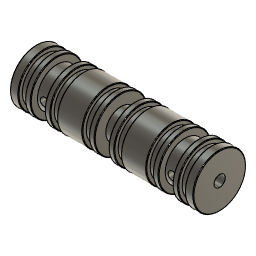
Timer ORings v3 (Autodesk Fusion 360 design; units mm, degrees)
Autodesk Fusion 360 part; units mm, degrees
sketch "Piston" plane through (0, 0, 0) normal (0, 1, 0) x (1, 0, 0)
  line L0 (0, 0) -> (0, -9.398)
  line L1 (0, -9.398) -> (1, -9.398)
  line L2 (1, -9.398) -> (2.5527, -9.398) construction
  line L3 (7.3876, -9.398) -> (7.3876, -7)
  line L4 (7.3876, -7) -> (12.3876, -7)
  line L5 (12.3876, -7) -> (12.3876, -9.398)
  line L6 (12.3876, -9.398) -> (14.3876, -9.398)
  line L7 (14.3876, -9.398) -> (14.3876, -7.9883)
  line L8 (14.3876, -7.9883) -> (16.7752, -7.9883)
  line L9 (16.7752, -7.9883) -> (16.7752, -9.398)
  line L10 (-1.3, -9.525) -> (30.7127, -9.525)
  line L11 (25.7752, -9.398) -> (25.7752, -7.9883)
  line L12 (25.7752, -7.9883) -> (28.1628, -7.9883)
  line L13 (28.1628, -7.9883) -> (28.1628, -9.398)
  line L14 (30.1628, -9.398) -> (30.1628, -5.398)
  line L15 (30.1628, -5.398) -> (32.6628, -5.398)
  line L16 (35.1628, -5.398) -> (35.1628, -9.398)
  line L17 (-1.7467, -7.9883) -> (1, -7.9883) construction
  line L18 (5.3876, -9.398) -> (5.3876, -7.9883)
  line L19 (5.3876, -7.9883) -> (3, -7.9883)
  line L20 (3, -7.9883) -> (3, -9.398)
  line L21 (32.6628, 7.102) -> (32.6628, -15.898)
  line L22 (16.7752, -9.398) -> (25.7752, -9.398)
  line L23 (28.1628, -9.398) -> (30.1628, -9.398)
  line L24 (5.3876, -9.398) -> (7.3876, -9.398)
  line L25 (3, -9.398) -> (0, -9.398)
  line L26 (32.6628, -5.398) -> (35.1628, -5.398)
  line L27 (0, 0) -> (32.6628, 0)
  line L28 (0, -2) -> (12, -2)
  line L29 (12, -2) -> (12, 0)
  dimension "d75" = 9.398
  dimension "d77" = 2.3876
  dimension "d78" = 9.525
  dimension "d79" = 2
  dimension "d80" = 5
  dimension "d81" = 9
  dimension "d82" = 2.3876
  dimension "d83" = 4
  dimension "d84" = 5
  dimension "d85" = 7.9883
  dimension "d86" = 2
  dimension "d87" = 2.3876
  dimension "d88" = 2
  dimension "d90" = 11.3876
  dimension "d91" = 3
  dimension "d92" = 2
  constraint coincident L0.start L27.start
  constraint vertical L0
  constraint perpendicular L0 L1
  constraint perpendicular L0 L2
  constraint coincident L2 L3.start
  constraint perpendicular L2 L3
  constraint perpendicular L3 L4
  constraint coincident L2 L5.end
  constraint perpendicular L2 L5
  constraint coincident L2 L6.end
  constraint perpendicular L6 L7
  constraint perpendicular L7 L8
  constraint coincident L2 L9.end
  constraint perpendicular L2 L9
  constraint parallel L2 L10
  constraint coincident L2 L11.start
  constraint perpendicular L2 L11
  constraint perpendicular L11 L12
  constraint coincident L2 L13.end
  constraint perpendicular L2 L13
  constraint coincident L2 L14.start
  constraint perpendicular L14 L15
  constraint coincident L2 L16.end
  constraint perpendicular L2 L16
  constraint perpendicular L5 L17
  constraint coincident L17 L18.end
  constraint perpendicular L17 L18
  constraint coincident L17 L19.end
  constraint perpendicular L2 L20
  constraint collinear L8 L17
  constraint perpendicular L2 L21
  constraint perpendicular L3 L24
  constraint perpendicular L0 L25
  constraint coincident L21 L15.end
  constraint perpendicular L14 L26
  constraint coincident L21 L27.end
  constraint perpendicular L21 L27
  constraint collinear L12 L17
  constraint coincident L0 L28.start
  constraint perpendicular L0 L28
  constraint coincident L27 L29.end
  constraint perpendicular L27 L29
  measures "d75" distance of L0.start L0.end
  measures "d77" distance of L7 L9
  measures "d78" distance of L0.start L10
  measures "d79" distance of L5 L7
  measures "d80" distance of L3 L5
  measures "d81" distance of L9 L11
  measures "d82" distance of L11 L13
  measures "d83" distance of L14.start L14.end
  measures "d84" distance of L14.end L16.start
  measures "d85" distance of L0.start L17
  measures "d86" distance of L3 L18
  measures "d87" distance of L18 L20
  measures "d88" distance of L13 L14
  measures "d90" distance of L7.end L19.end
  measures "d91" distance of L0 L20
  measures "d92" distance of L27 L28
revolve "Revolve3" add sketch "Piston" angle 360 about axis through (0, 0, 0) along (1, 0, 0) contours L0 L1 L3 L4 L5 L6 L7 L8 L9 L11 L12 L13 L14 L15 L18 L19 L20 L21 L22 L23 L24 L25 L27 L28 L29 makes body 1
sketch "Sketch6" plane through (0, 0, 0) normal (0, 1, 0) x (1, 0, 0)
  line L0 (7.3876, -7) -> (12.3876, -7)
  circle A0 centre (9.8876, 0) radius 1.5
  line L1 (9.8876, -19.5) -> (9.8876, 5.5) construction
  dimension "d96" = 3
  constraint vertical L1
  constraint midpoint L0 L1
  constraint coincident A0.centre L1
  measures "d96" diameter of A0
extrude "Extrude15" cut sketch "Sketch6" along normal through all and the other way through all bodies 1
mirror "Mirror1" about plane through (32.6628, 0, 0) normal (1, 0, 0) of bodies 1 makes body 2
combine "Combine3" operation add target body 1 tool bodies 2
fillet "Fillet2" radius 0.2 20 edges at (0, -3.3985, -8.762) (3, -3.3985, -8.762) (5.3876, -3.3985, -8.762) (7.3876, -3.3985, -8.762) (12.3876, -3.3985, -8.762) (14.3876, -3.3985, -8.762) (16.7752, -3.3985, -8.762) (25.7752, -3.3985, -8.762) (28.1628, -3.3985, -8.762) (37.1628, -3.3985, -8.762) (35.1628, -3.3985, -8.762) (30.1628, -3.3985, -8.762) (39.5504, -3.3985, -8.762) (48.5504, -3.3985, -8.762) (50.938, -3.3985, -8.762) (52.938, -3.3985, -8.762) (57.938, -3.3985, -8.762) (59.938, -3.3985, -8.762) (62.3256, -3.3985, -8.762) (65.3256, -3.3985, -8.762) on bodies 1
equation "d8 = 0.747 in / 2"
equation "d10 = d8"
equation "d75 = 0.740 in / 2"
equation "d78 = 0.75 in / 2"
equation "d81 = d79 * 2 + d80"
equation "d82 = d77"
equation "d84 = d80"
equation "d85 = 0.629 in / 2"
equation "d86 = d79"
equation "d87 = d77"
equation "d88 = d79"
